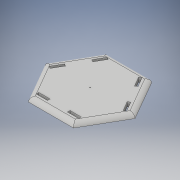
# Autodesk Inventor part: Bot_
Saved by Autodesk Inventor 2019.4 (Build 234330000, 330)
## iProperties
Created: 2020-04-07
Part Number: Bot_
Material: Generic
Document SubType Name: Modeling
Designer: Jorian Brusind
Density: 1 g/cm^3
Appearance: Default
Author: Jorian Brusind
Autodesk Inventor part; units mm, degrees
ref_plane "YZ Plane" through (0, 0, 0) normal (1, 0, 0) x (0, 1, 0)
ref_plane "XZ Plane" through (0, 0, 0) normal (0, 1, 0) x (-1, 0, 0)
ref_plane "XY Plane" through (0, 0, 0) normal (0, 0, 1) x (1, 0, 0)
sketch "Sketch1" plane through (0, 0, 0) normal (0, 1, 0) x (-1, 0, 0)
  line L0 (51.9615, 0) -> (25.9808, -45)
  line L1 (25.9808, -45) -> (-25.9808, -45)
  line L2 (-25.9808, -45) -> (-51.9615, 0)
  line L3 (-51.9615, 0) -> (-25.9808, 45)
  line L4 (-25.9808, 45) -> (25.9808, 45)
  line L5 (25.9808, 45) -> (51.9615, 0)
  point P0 (0, 0)
  point P1 (0, 0)
  dimension "d1" = 45
  dimension "d2" = 45
  constraints: 12 end point, 1 coincident, 13 other
  measures "d1" distance from line of L1 point (0, 0)
  measures "d2" vertical distance of L4.end L0.start
extrude "Extrusion1" add sketch "Sketch1" along normal blind 5
sketch "Sketch2" plane through (0, 5, 0) normal (0, 1, 0) x (1, 0, 0)
  line L0 (-25.9808, 45) -> (-51.9615, 0) projected
  line L1 (-38.9711, 22.5) -> (-47.9711, 6.9115)
  line L2 (-38.9711, 22.5) -> (-29.9711, 38.0885)
  line L3 (-47.9711, 6.9115) -> (-40.1769, 2.4115)
  line L4 (-38.226, 8.7907) -> (-44.726, -2.4676)
  line L5 (-44.726, -2.4676) -> (-42.1279, -3.9676)
  line L6 (-42.1279, -3.9676) -> (-35.6279, 7.2907)
  line L7 (-35.6279, 7.2907) -> (-38.226, 8.7907)
  line L8 (-38.226, 8.7907) -> (-42.1279, -3.9676) construction
  line L9 (-44.726, -2.4676) -> (-35.6279, 7.2907) construction
  line L10 (-38.226, 8.7907) -> (-25.226, 8.7907) construction
  line L11 (-29.9711, 38.0885) -> (-22.1769, 33.5885)
  line L12 (-17.6279, 38.4676) -> (-24.1279, 27.2093)
  line L13 (-24.1279, 27.2093) -> (-26.726, 28.7093)
  line L14 (-26.726, 28.7093) -> (-20.226, 39.9676)
  line L15 (-20.226, 39.9676) -> (-17.6279, 38.4676)
  line L16 (-17.6279, 38.4676) -> (-26.726, 28.7093) construction
  line L17 (-24.1279, 27.2093) -> (-20.226, 39.9676) construction
  circle A0 centre (0, 0) radius 0.5
  dimension "d5" = 18
  dimension "d6" = 18
  dimension "d7" = 9
  dimension "d8" = 90
  dimension "d9" = 13
  dimension "d10" = 120
  dimension "d11" = 3
  dimension "d12" = 9
  dimension "d13" = 13
  dimension "d14" = 3
  dimension "d15" = 90
  dimension "d16" = 1
  constraints: 34 end point, 5 midpoint, 4 parallel, 4 perpendicular, 2 point on line, 1 centre point, 1 coincident, 1 equal length, 1 horizontal
  measures "d5" distance of L1.start L1.end
  measures "d6" distance of L1.start L2.end
  measures "d7" distance of L1.end L3.end
  measures "d8" angle of L0 L3
  measures "d9" distance of L4.start L4.end
  measures "d10" angle of L4 L10
  measures "d11" distance of L5.end L4.end
  measures "d12" distance of L2.end L11.end
  measures "d13" distance of L12.start L12.end
  measures "d14" distance of L12.end L13.end
  measures "d15" angle of L11 L14
  measures "d16" diameter of A0
extrude "Extrusion2" cut sketch "Sketch2" against normal blind 5
pattern_circular "Circular Pattern1" count 3 over 360 about axis through (0, 5, 0) along (0, -1, 0) of "Extrusion2"
fillet "Fillet1" radius 5 6 edges at (38.9711, 5, 22.5) (38.9711, 5, -22.5) (0, 5, -45) (-38.9711, 5, -22.5) (-38.9711, 5, 22.5) (0, 5, 45)
body "Solid1"
